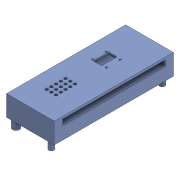
# Autodesk Inventor part: podstawa_2
Saved by Autodesk Inventor 2021 (Build 250183000, 183)
## iProperties
Created: 2022-06-23
Part Number: podstawa_2
Material: Generic
Document SubType Name: Modeling
Designer: agnpi
Density: 1 g/cm^3
Appearance: Orange
Author: agnpi
Autodesk Inventor part; units mm, degrees
ref_plane "YZ Plane" through (0, 0, 0) normal (1, 0, 0) x (0, 1, 0)
ref_plane "XZ Plane" through (0, 0, 0) normal (0, 1, 0) x (-1, 0, 0)
ref_plane "XY Plane" through (0, 0, 0) normal (0, 0, 1) x (1, 0, 0)
sketch "Sketch1" plane through (0, 0, 0) normal (0, 1, 0) x (-1, 0, 0)
  line L0 (62.2, 0) -> (-72.2, 0) projected
  line L1 (0, -144.2) -> (0, 144.2) projected
  line L2 (-35, 95) -> (35, 95)
  line L3 (35, 95) -> (35, -95)
  line L4 (35, -95) -> (-35, -95)
  line L5 (-35, -95) -> (-35, 95)
  line L6 (-35, 95) -> (35, -95) construction
  line L7 (35, 95) -> (-35, -95) construction
  line L8 (-53, 103) -> (43, 103)
  line L9 (43, 103) -> (43, -103)
  line L10 (43, -103) -> (-53, -103)
  line L11 (-53, -103) -> (-53, 103)
  point P0 (0, 0)
  dimension "d0" = 70
  dimension "d1" = 190
  dimension "d2" = 8
  dimension "d3" = 8
  dimension "d4" = 18
  dimension "d5" = 8
  constraints: 20 end point, 3 parallel, 3 perpendicular, 2 horizontal, 2 midpoint
  measures "d0" distance of L3.end L4.end
  measures "d1" distance of L2.end L3.end
  measures "d2" distance between parallel lines of L2 L8
  measures "d3" distance between parallel lines of L10 L4
  measures "d4" distance between parallel lines of L11 L5
  measures "d5" distance between parallel lines of L9 L3
extrude "Extrusion1" add sketch "Sketch1" along normal blind 8 contours L3 L4 L1 L0 | L0 L1 L2 L3 | L1 L4 L5 L0 | L0 L5 L2 L1
extrude "Extrusion2" add sketch "Sketch1" along normal blind 80 contours L9 L10 L1 L4 L3 L0 | L0 L3 L2 L1 L8 L9 | L1 L2 L5 L0 L11 L8 | L10 L11 L0 L5 L4 L1
move faces "Move1" translate (-16, 0, 0) faces at (35, 32, -31.6667)
move faces "Move5" translate (-8, 0, 0) faces at (53, 53.3333, 34.3333)
move faces "Move6" translate (-8, 0, 0) faces at (45, 26.6667, 34.3333)
move faces "Move7" translate (0, 0, -8) faces at (-17, 56, 95)
move faces "Move8" translate (0, 0, -8) faces at (-16.3333, 26.6667, 103)
move faces "Move9" translate (0, 0, -8) faces at (-17, 56, 87)
move faces "Move10" translate (0, 0, -8) faces at (-16.3333, 26.6667, 95)
thicken "Thicken1" operation add thickness 3 both sides no extend neighbours yes toward (0, 0, 1) faces at (-16.3333, 26.6667, 87)
thicken "Thicken3" operation add thickness 3 both sides no extend neighbours yes toward (0, 0, -1) faces at (10.3333, 26.6667, -103)
thicken "Thicken4" operation add thickness 1 both sides no extend neighbours yes toward (1, 0, 0) faces at (-35, 56, -37)
thicken "Thicken5" operation add thickness 1 both sides no extend neighbours yes toward (-1, 0, 0) faces at (19, 56, 21)
sketch "Sketch6" plane through (0, 0, 0) normal (0, -1, 0) x (1, 0, 0)
  line L0 (37, 90) -> (37, -106) projected
  line L1 (37, -106) -> (-43, -106) projected
  line L2 (37, 90) -> (-43, 90)
  line L3 (-43, 90) -> (-43, -106)
  line L4 (-43, -106) -> (37, -106)
  line L5 (37, -106) -> (37, 90)
  point P0 (0, 0)
  constraints: 8 end point, 2 parallel, 1 horizontal, 1 perpendicular
extrude "Extrusion7" cut sketch "Sketch6" against normal blind 45
sketch "Sketch10" plane through (-34, 80, 79) normal (1, 0, 0) x (0, 0, -1)
  line L0 (0, 0) -> (174, 0) projected
  line L1 (0, 0) -> (174, 0)
  line L2 (174, 0) -> (174, -4)
  line L3 (174, -4) -> (0, -4)
  line L4 (0, -4) -> (0, 0)
  line L5 (174, -35) -> (174, 0) projected
  point P0 (79, -80)
  point P1 (174, -6.75)
  point P2 (174, -13.5)
  dimension "d101" = 4
  constraints: 8 end point, 2 parallel, 2 point on line, 1 horizontal, 1 perpendicular
  measures "d101" distance between parallel lines of L0 L3
extrude "Extrusion10" add sketch "Sketch10" along normal up to surface (52 mm away)
sketch "Sketch11" plane through (0, 80, 0) normal (0, 1, 0) x (1, 0, 0)
  line L0 (18, 90) -> (-24, 90)
  line L1 (-24, 90) -> (-24, -74)
  line L2 (-24, -74) -> (18, -74)
  line L3 (18, -74) -> (18, 90)
  line L4 (37, -90) -> (37, 106) projected
  line L5 (37, 106) -> (-43, 106) projected
  line L6 (-43, -90) -> (37, -90) projected
  line L7 (-43, 106) -> (-43, -90) projected
  point P0 (0, 0)
  dimension "d104" = 19
  dimension "d105" = 16
  dimension "d106" = 16
  dimension "d107" = 19
  constraints: 8 end point, 2 parallel, 1 horizontal, 1 perpendicular
  measures "d104" distance between parallel lines of L4 L3
  measures "d105" distance between parallel lines of L5 L0
  measures "d106" distance between parallel lines of L6 L2
  measures "d107" distance between parallel lines of L7 L1
extrude "Extrusion11" cut sketch "Sketch11" against normal blind 8 contours L3 L2 L1 L0
sketch "Sketch13" plane through (-24, 80, 74) normal (1, 0, 0) x (0, 0, -1)
  line L0 (0, 0) -> (164, 0) projected
  line L1 (164, -4) -> (0, -4) projected
  line L2 (0, 0) -> (164, 0)
  line L3 (164, 0) -> (164, -4)
  line L4 (164, -4) -> (0, -4)
  line L5 (0, -4) -> (0, 0)
  point P0 (74, -80)
  point P1 (0, -4)
  constraints: 8 end point, 2 parallel, 1 horizontal, 1 perpendicular
extrude "Extrusion13" add sketch "Sketch13" along normal up to surface (42 mm away)
sketch "Sketch14" plane through (37, 80, 90) normal (1, 0, 0) x (0, 0, -1)
  line L0 (11, -35) -> (11, -4) projected
  line L1 (11, -4) -> (185, -4)
  line L2 (185, -4) -> (185, -13.5)
  line L3 (185, -13.5) -> (11, -13.5)
  line L4 (11, -13.5) -> (11, -4)
  line L5 (0, 0) -> (196, 0) projected
  point P0 (90, -80)
  point P1 (11, -13.5)
  dimension "d114" = 174
  dimension "d115" = 4
  dimension "d116" = 9.5
  constraints: 8 end point, 2 parallel, 1 horizontal, 1 perpendicular, 1 point on line
  measures "d114" distance of L2.end L3.end
  measures "d115" distance between parallel lines of L5 L1
  measures "d116" distance between parallel lines of L3 L1
extrude "Extrusion14" cut sketch "Sketch14" against normal blind 8
sketch "Sketch17" plane through (0, 45, 0) normal (0, -1, 0) x (1, 0, 0)
  point P0 (0, 0)
move faces "Move11" translate (-1, 0, 0) faces at (-43, 56.6667, -40.6667)
move faces "Move12" translate (0, 0, -3) faces at (-16.6667, 65.6667, 79)
move faces "Move13" translate (0, 0, 3) faces at (0.6667, 65.6667, -95)
move faces "Move14" translate (0, 0, 3) faces at (-17, 56.6667, 90)
move faces "Move15" translate (0, 0, -3) faces at (10, 68.3333, -106)
move faces "Move16" translate (0, 0, 3) faces at (-16.6667, 65.6667, 76) (10, 80, 25.6667)
move faces "Move17" translate (0, 0, -3) faces at (0.6667, 65.6667, -92)
sketch "Sketch23" plane through (0, 45, 0) normal (0, -1, 0) x (1, 0, 0)
  line L0 (-34, 79) -> (18, 79) projected
  line L1 (-29.343, 79) -> (-34, 74.343)
  line L2 (-34, -95) -> (-34, 79) projected
  line L3 (-34, -90.343) -> (-29.343, -95)
  line L4 (-34, -95) -> (18, -95) projected
  point P0 (0, 0)
  dimension "d178" = 45
  dimension "d179" = 6.586
  dimension "d180" = 45
  dimension "d181" = 6.586
  constraints: 4 end point, 4 point on line
  measures "d178" angle of L2 L1
  measures "d179" distance of L1.start L1.end
  measures "d180" angle of L4 L3
  measures "d181" distance of L3.start L3.end
extrude "Extrusion20" add sketch "Sketch23" against normal up to surface (31 mm away)
sketch "Sketch24" plane through (0, 45, 0) normal (0, -1, 0) x (1, 0, 0)
  circle A0 centre (-36, 85) radius 6
  circle A1 centre (-36, -101) radius 6
  line L0 (-44, -109) -> (-44, 93) projected
  line L1 (-44, 93) -> (37, 93) projected
  line L2 (37, -109) -> (-44, -109) projected
  point P0 (0, 0)
  dimension "d184" = 12
  dimension "d185" = 12
  dimension "d186" = 8
  dimension "d187" = 8
  dimension "d188" = 8
  dimension "d189" = 8
  constraints: 2 centre point
  measures "d184" diameter of A0
  measures "d185" diameter of A1
  measures "d186" distance from line of L0 A0.centre
  measures "d187" distance from line of L1 A0.centre
  measures "d188" distance from line of L2 A1.centre
  measures "d189" distance from line of L0 A1.centre
extrude "Extrusion21" add sketch "Sketch24" along normal blind 15
sketch "Sketch27" plane through (18, 76, -95) normal (0, -1, 0) x (1, 0, 0)
  line L0 (-37, 40) -> (-17.8, 40)
  line L1 (-17.8, 40) -> (-17.8, 67)
  line L2 (-17.8, 67) -> (-37, 67)
  line L3 (-37, 67) -> (-37, 40)
  line L4 (-52, 169.343) -> (-52, 4.657) projected
  line L5 (-47.343, 0) -> (0, 0) projected
  point P0 (-18, 95)
  dimension "d202" = 19.2
  dimension "d203" = 27
  dimension "d204" = 15
  dimension "d205" = 40
  constraints: 8 end point, 2 parallel, 1 horizontal, 1 perpendicular
  measures "d202" distance of L2.end L1.end
  measures "d203" distance of L1.end L0.end
  measures "d204" distance between parallel lines of L3 L4
  measures "d205" distance between parallel lines of L5 L0
extrude "Extrusion23" cut sketch "Sketch27" against normal blind 1.505
sketch "Sketch28" plane through (18, 76, -95) normal (0, -1, 0) x (1, 0, 0)
  line L0 (-41, 39.3) -> (-13.6, 39.3)
  line L1 (-13.6, 39.3) -> (-13.6, 67.7)
  line L2 (-13.6, 67.7) -> (-41, 67.7)
  line L3 (-41, 67.7) -> (-41, 39.3)
  line L4 (-40.15, 41.45) -> (-40.15, 42.55)
  line L5 (-37.95, 41.45) -> (-37.95, 42.75)
  arc A0 (-37.95, 42.75) -> (-40.15, 42.55) centre (-39.0409, 42.55) ccw
  arc A1 (-40.15, 41.45) -> (-37.95, 41.45) centre (-39.05, 41.45) ccw
  arc A2 (-40.15, 64.45) -> (-37.95, 64.45) centre (-39.05, 64.45) ccw
  line L6 (-40.15, 64.45) -> (-40.15, 65.55)
  arc A3 (-37.95, 65.75) -> (-40.15, 65.55) centre (-39.0409, 65.55) ccw
  line L7 (-37.95, 64.45) -> (-37.95, 65.75)
  arc A4 (-16.65, 41.45) -> (-14.45, 41.45) centre (-15.55, 41.45) ccw
  line L8 (-16.65, 41.45) -> (-16.65, 42.55)
  arc A5 (-14.45, 42.75) -> (-16.65, 42.55) centre (-15.5409, 42.55) ccw
  line L9 (-14.45, 41.45) -> (-14.45, 42.75)
  arc A6 (-16.65, 64.45) -> (-14.45, 64.45) centre (-15.55, 64.45) ccw
  line L10 (-16.65, 64.45) -> (-16.65, 65.55)
  arc A7 (-14.45, 65.75) -> (-16.65, 65.55) centre (-15.5409, 65.55) ccw
  line L11 (-14.45, 64.45) -> (-14.45, 65.75)
  line L12 (-40.9, 48.1) -> (-38.1, 48.1)
  line L13 (-38.1, 48.1) -> (-38.1, 58.9)
  line L14 (-38.1, 58.9) -> (-40.9, 58.9)
  line L15 (-40.9, 58.9) -> (-40.9, 48.1)
  line L16 (-37, 40) -> (-37, 67) projected
  line L17 (-37, 67) -> (-17.8, 67) projected
  point P0 (-18, 95)
  dimension "d208" = 27.4
  dimension "d209" = 28.4
  dimension "d218" = 1.1
  dimension "d219" = 2.2
  dimension "d221" = 1.3
  dimension "d223" = 1.1
  dimension "d227" = 23
  dimension "d230" = 23.5
  dimension "d236" = 10.8
  dimension "d272" = 2.8
  dimension "d273" = 1.1
  dimension "d275" = 2.15
  dimension "d276" = 24.5
  dimension "d277" = 8.8
  dimension "d278" = 1.1
  dimension "d279" = 0.7
  dimension "d282" = 21.45
  constraints: 32 end point, 16 point on circle, 8 centre point, 4 parallel, 3 horizontal, 3 vertical, 2 perpendicular, 1 tangent, 30 other
  measures "d208" distance of L2.end L1.end
  measures "d209" distance of L1.end L0.end
  measures "d218" distance of L4.start L4.end
  measures "d219" distance of L5.start L4.start
  measures "d221" distance of L5.end L5.start
  measures "d223" radius of A1
  measures "d227" distance of A1.centre A2.centre
  measures "d230" distance of A1.centre A4.centre
  measures "d236" distance of L13.end L12.end
  measures "d272" distance between parallel lines of L13 L15
  measures "d273" vertical distance of A3.centre A2.centre
  measures "d275" distance from line of L0 A1.centre
  measures "d276" distance between parallel lines of L1 L13
  measures "d277" distance between parallel lines of L0 L12
  measures "d278" distance between parallel lines of L16 L13
  measures "d279" distance between parallel lines of L2 L17
  measures "d282" distance from line of L16 A6.centre
extrude "Extrusion25" cut sketch "Sketch28" against normal through all contours L4 A0 L5 A1 | L6 A3 L7 A2 | L8 A5 L9 A4 | L10 A7 L11 A6
extrude "Extrusion27" cut sketch "Sketch28" against normal blind 2 contours L15 L14 L13 L12
sketch "Sketch31" plane through (0, 45, 0) normal (0, -1, 0) x (1, 0, 0)
  circle A0 centre (25, 86) radius 4.5
  circle A1 centre (25, -102) radius 4.5
  line L0 (37, -109) -> (-44, -109) projected
  line L1 (-44, 93) -> (37, 93) projected
  line L2 (37, 93) -> (37, -109) projected
  point P0 (0, 0)
  dimension "d243" = 9
  dimension "d244" = 9
  dimension "d245" = 7
  dimension "d246" = 7
  dimension "d247" = 12
  dimension "d248" = 12
  constraints: 2 centre point
  measures "d243" diameter of A0
  measures "d244" diameter of A1
  measures "d245" distance from line of L0 A1.centre
  measures "d246" distance from line of L1 A0.centre
  measures "d247" distance from line of L2 A0.centre
  measures "d248" distance from line of L2 A1.centre
extrude "Extrusion28" add sketch "Sketch31" along normal blind 15
sketch "Sketch32" plane through (18, 76, -95) normal (0, -1, 0) x (1, 0, 0)
  line L0 (-11, 153) -> (-41, 153)
  line L1 (-41, 153) -> (-41, 111)
  line L2 (-41, 111) -> (-11, 111)
  line L3 (-11, 111) -> (-11, 153)
  line L4 (0, 0) -> (0, 174) projected
  line L5 (0, 174) -> (-47.343, 174) projected
  line L6 (-20.1651, 149.25) -> (-18, 150.5)
  line L7 (-18, 150.5) -> (-15.8349, 149.25)
  line L8 (-15.8349, 149.25) -> (-15.8349, 146.75)
  line L9 (-15.8349, 146.75) -> (-18, 145.5)
  line L10 (-18, 145.5) -> (-20.1651, 146.75)
  line L11 (-20.1651, 146.75) -> (-20.1651, 149.25)
  line L12 (-18, 142.5) -> (-15.8349, 141.25)
  line L13 (-15.8349, 141.25) -> (-15.8349, 138.75)
  line L14 (-15.8349, 138.75) -> (-18, 137.5)
  line L15 (-18, 137.5) -> (-20.1651, 138.75)
  line L16 (-20.1651, 138.75) -> (-20.1651, 141.25)
  line L17 (-20.1651, 141.25) -> (-18, 142.5)
  line L18 (-18, 134.5) -> (-15.8349, 133.25)
  line L19 (-15.8349, 133.25) -> (-15.8349, 130.75)
  line L20 (-15.8349, 130.75) -> (-18, 129.5)
  line L21 (-18, 129.5) -> (-20.1651, 130.75)
  line L22 (-20.1651, 130.75) -> (-20.1651, 133.25)
  line L23 (-20.1651, 133.25) -> (-18, 134.5)
  line L24 (-18, 126.5) -> (-15.8349, 125.25)
  line L25 (-15.8349, 125.25) -> (-15.8349, 122.75)
  line L26 (-15.8349, 122.75) -> (-18, 121.5)
  line L27 (-18, 121.5) -> (-20.1651, 122.75)
  line L28 (-20.1651, 122.75) -> (-20.1651, 125.25)
  line L29 (-20.1651, 125.25) -> (-18, 126.5)
  line L30 (-18, 118.5) -> (-15.8349, 117.25)
  line L31 (-15.8349, 117.25) -> (-15.8349, 114.75)
  line L32 (-15.8349, 114.75) -> (-18, 113.5)
  line L33 (-18, 113.5) -> (-20.1651, 114.75)
  line L34 (-20.1651, 114.75) -> (-20.1651, 117.25)
  line L35 (-20.1651, 117.25) -> (-18, 118.5)
  line L36 (-26, 150.5) -> (-23.8349, 149.25)
  line L37 (-23.8349, 149.25) -> (-23.8349, 146.75)
  line L38 (-23.8349, 146.75) -> (-26, 145.5)
  line L39 (-26, 145.5) -> (-28.1651, 146.75)
  line L40 (-28.1651, 146.75) -> (-28.1651, 149.25)
  line L41 (-28.1651, 149.25) -> (-26, 150.5)
  line L42 (-26, 142.5) -> (-23.8349, 141.25)
  line L43 (-23.8349, 141.25) -> (-23.8349, 138.75)
  line L44 (-23.8349, 138.75) -> (-26, 137.5)
  line L45 (-26, 137.5) -> (-28.1651, 138.75)
  line L46 (-28.1651, 138.75) -> (-28.1651, 141.25)
  line L47 (-28.1651, 141.25) -> (-26, 142.5)
  line L48 (-26, 134.5) -> (-23.8349, 133.25)
  line L49 (-23.8349, 133.25) -> (-23.8349, 130.75)
  line L50 (-23.8349, 130.75) -> (-26, 129.5)
  line L51 (-26, 129.5) -> (-28.1651, 130.75)
  line L52 (-28.1651, 130.75) -> (-28.1651, 133.25)
  line L53 (-28.1651, 133.25) -> (-26, 134.5)
  line L54 (-26, 126.5) -> (-23.8349, 125.25)
  line L55 (-23.8349, 125.25) -> (-23.8349, 122.75)
  line L56 (-23.8349, 122.75) -> (-26, 121.5)
  line L57 (-26, 121.5) -> (-28.1651, 122.75)
  line L58 (-28.1651, 122.75) -> (-28.1651, 125.25)
  line L59 (-28.1651, 125.25) -> (-26, 126.5)
  line L60 (-26, 118.5) -> (-23.8349, 117.25)
  line L61 (-23.8349, 117.25) -> (-23.8349, 114.75)
  line L62 (-23.8349, 114.75) -> (-26, 113.5)
  line L63 (-26, 113.5) -> (-28.1651, 114.75)
  line L64 (-28.1651, 114.75) -> (-28.1651, 117.25)
  line L65 (-28.1651, 117.25) -> (-26, 118.5)
  line L66 (-34, 150.5) -> (-31.8349, 149.25)
  line L67 (-31.8349, 149.25) -> (-31.8349, 146.75)
  line L68 (-31.8349, 146.75) -> (-34, 145.5)
  line L69 (-34, 145.5) -> (-36.1651, 146.75)
  line L70 (-36.1651, 146.75) -> (-36.1651, 149.25)
  line L71 (-36.1651, 149.25) -> (-34, 150.5)
  line L72 (-34, 142.5) -> (-31.8349, 141.25)
  line L73 (-31.8349, 141.25) -> (-31.8349, 138.75)
  line L74 (-31.8349, 138.75) -> (-34, 137.5)
  line L75 (-34, 137.5) -> (-36.1651, 138.75)
  line L76 (-36.1651, 138.75) -> (-36.1651, 141.25)
  line L77 (-36.1651, 141.25) -> (-34, 142.5)
  line L78 (-34, 134.5) -> (-31.8349, 133.25)
  line L79 (-31.8349, 133.25) -> (-31.8349, 130.75)
  line L80 (-31.8349, 130.75) -> (-34, 129.5)
  line L81 (-34, 129.5) -> (-36.1651, 130.75)
  line L82 (-36.1651, 130.75) -> (-36.1651, 133.25)
  line L83 (-36.1651, 133.25) -> (-34, 134.5)
  line L84 (-34, 126.5) -> (-31.8349, 125.25)
  line L85 (-31.8349, 125.25) -> (-31.8349, 122.75)
  line L86 (-31.8349, 122.75) -> (-34, 121.5)
  line L87 (-34, 121.5) -> (-36.1651, 122.75)
  line L88 (-36.1651, 122.75) -> (-36.1651, 125.25)
  line L89 (-36.1651, 125.25) -> (-34, 126.5)
  line L90 (-34, 118.5) -> (-31.8349, 117.25)
  line L91 (-31.8349, 117.25) -> (-31.8349, 114.75)
  line L92 (-31.8349, 114.75) -> (-34, 113.5)
  line L93 (-34, 113.5) -> (-36.1651, 114.75)
  line L94 (-36.1651, 114.75) -> (-36.1651, 117.25)
  line L95 (-36.1651, 117.25) -> (-34, 118.5)
  point P0 (-18, 95)
  point P1 (-18, 148)
  dimension "d251" = 42
  dimension "d252" = 30
  dimension "d253" = 11
  dimension "d254" = 21
  dimension "d255" = 2.5
  dimension "d256" = 7
  dimension "d257" = 5
  dimension "d259" = 2.5
  dimension "d262" = 8
  dimension "d265" = 8
  constraints: 188 end point, 2 horizontal, 2 parallel, 1 perpendicular, 1 vertical, 181 other
  measures "d251" distance of L2.end L0.start
  measures "d252" distance between parallel lines of L1 L3
  measures "d253" distance between parallel lines of L4 L3
  measures "d254" distance between parallel lines of L5 L0
  measures "d255" distance of L8.end L7.end
  measures "d256" distance from line of L3 point (-18, 148)
  measures "d257" distance from line of L0 point (-18, 148)
  measures "d259" distance of L9.end L10.end
  measures "d262" distance of L6.end L12.start
  measures "d265" distance of L6.end L36.start
extrude "Extrusion29" cut sketch "Sketch32" against normal through all contours L6 L7 L8 L9 L10 L11 | L12 L13 L14 L15 L16 L17 | L18 L19 L20 L21 L22 L23 | L24 L25 L26 L27 L28 L29 | L30 L31 L32 L33 L34 L35 | L36 L37 L38 L39 L40 L41 | L42 L43 L44 L45 L46 L47 | L48 L49 L50 L51 L52 L53 | L54 L55 L56 L57 L58 L59 | L60 L61 L62 L63 L64 L65 | L66 L67 L68 L69 L70 L71 | L72 L73 L74 L75 L76 L77 | L78 L79 L80 L81 L82 L83 | L84 L85 L86 L87 L88 L89 | L90 L91 L92 L93 L94 L95
sketch "Sketch33" plane through (18, 77.505, -95) normal (0, -1, 0) x (1, 0, 0)
  line L0 (-22.25, 66.5) -> (-36.5, 66.5)
  line L1 (-36.5, 66.5) -> (-36.5, 40.5)
  line L2 (-36.5, 40.5) -> (-22.25, 40.5)
  line L3 (-22.25, 40.5) -> (-22.25, 66.5)
  line L4 (-37, 40) -> (-37, 67) projected
  line L5 (-37, 67) -> (-17.8, 67) projected
  point P0 (-18, 95)
  dimension "d283" = 26
  dimension "d284" = 14.25
  dimension "d287" = 0.5
  dimension "d288" = 0.5
  constraints: 8 end point, 2 parallel, 1 horizontal, 1 perpendicular
  measures "d283" distance of L0.end L1.end
  measures "d284" distance between parallel lines of L1 L3
  measures "d287" distance between parallel lines of L5 L0
  measures "d288" distance between parallel lines of L1 L4
extrude "Extrusion30" cut sketch "Sketch33" against normal through all
body "Solid1"
